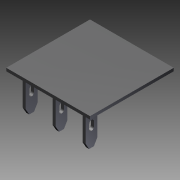
# Autodesk Inventor part: UB216KKW015C-NR
Saved by Autodesk Inventor 2015 SP1 (Build 190203100, 203)
## iProperties
Category: Electrical
Company: Autodesk Inc.
Created: 2014-12-16
Part Number: UB216KKW015C-NR
Catalog Web Link: http://www.nkkswitches.com/
Description: PC and Snap-in Mount Non-Illuminated Pushbuttons_ni_pole-Non-Illuminated Pushbuttons - Series UB2
Vendor: NKK Switches
Document SubType Name: Modeling
Designer: Autodesk Inc.
Manufacturer: NKKSWITCHES
Mass: 0.118482 g
Surface Area: 5.18676 cm^2
Volume: 0.118482 cm^3
Density: 1 g/cm^3
Material: Generic
Appearance: PSOLRGB-191-191-191
Title: UB21W01-5Cni_pole
Author: Autodesk Inc.
Comments: Non-Illuminated Pushbuttons - Series UB2
Autodesk Inventor part; units mm, degrees
sketch "Sketch_1" plane through (0, 0, 0) normal (0, 1, 0) x (-1, 0, 0)
  line L0 (7.112, -7.112) -> (7.112, 7.112)
  line L1 (7.112, 7.112) -> (-7.112, 7.112)
  line L2 (-7.112, 7.112) -> (-7.112, -7.112)
  line L3 (-7.112, -7.112) -> (7.112, -7.112)
  constraints: 8 end point
extrude "Extrusion1" add sketch "Sketch_1" along normal blind 0.508
sketch "Sketch_2" plane through (-5.08, 0, 0) normal (1, 0, 0) x (0, 0, -1)
  line L0 (-6.0833, -4.9859) -> (-5.4864, -6.0198)
  line L1 (-5.4864, -6.0198) -> (-4.6736, -6.0198)
  line L2 (-4.6736, -6.0198) -> (-4.0767, -4.9859)
  line L3 (-4.0767, -4.9859) -> (-4.0767, 0.508)
  line L4 (-4.0767, 0.508) -> (-6.0833, 0.508)
  line L5 (-6.0833, 0.508) -> (-6.0833, -4.9859)
  line L6 (-5.4864, -2.3622) -> (-5.4864, -3.1496)
  arc A0 (-5.4864, -3.1496) -> (-5.08, -3.556) centre (-5.08, -3.1496) ccw
  arc A1 (-5.08, -3.556) -> (-4.6736, -3.1496) centre (-5.08, -3.1496) ccw
  line L7 (-4.6736, -3.1496) -> (-4.6736, -2.3622)
  arc A2 (-4.6736, -2.3622) -> (-5.08, -1.9558) centre (-5.08, -2.3622) ccw
  arc A3 (-5.08, -1.9558) -> (-5.4864, -2.3622) centre (-5.08, -2.3622) ccw
  constraints: 16 end point, 8 point on circle, 4 centre point
extrude "Extrusion2" add sketch "Sketch_2" along normal mid plane 0.508
sketch "Sketch_4" plane through (0, 0, 0) normal (1, 0, 0) x (0, 1, 0)
  line L0 (-4.9859, 6.0833) -> (-6.0198, 5.4864)
  line L1 (-6.0198, 5.4864) -> (-6.0198, 4.6736)
  line L2 (-6.0198, 4.6736) -> (-4.9859, 4.0767)
  line L3 (-4.9859, 4.0767) -> (0.508, 4.0767)
  line L4 (0.508, 4.0767) -> (0.508, 6.0833)
  line L5 (0.508, 6.0833) -> (-4.9859, 6.0833)
  line L6 (-2.3622, 5.4864) -> (-3.1496, 5.4864)
  arc A0 (-3.1496, 5.4864) -> (-3.556, 5.08) centre (-3.1496, 5.08) ccw
  arc A1 (-3.556, 5.08) -> (-3.1496, 4.6736) centre (-3.1496, 5.08) ccw
  line L7 (-3.1496, 4.6736) -> (-2.3622, 4.6736)
  arc A2 (-2.3622, 4.6736) -> (-1.9558, 5.08) centre (-2.3622, 5.08) ccw
  arc A3 (-1.9558, 5.08) -> (-2.3622, 5.4864) centre (-2.3622, 5.08) ccw
  constraints: 16 end point, 8 point on circle, 4 centre point
extrude "Extrusion3" add sketch "Sketch_4" along normal mid plane 0.508
sketch "Sketch_6" plane through (5.08, 0, 0) normal (1, 0, 0) x (0, 0, -1)
  line L0 (-6.0833, -4.9859) -> (-5.4864, -6.0198)
  line L1 (-5.4864, -6.0198) -> (-4.6736, -6.0198)
  line L2 (-4.6736, -6.0198) -> (-4.0767, -4.9859)
  line L3 (-4.0767, -4.9859) -> (-4.0767, 0.508)
  line L4 (-4.0767, 0.508) -> (-6.0833, 0.508)
  line L5 (-6.0833, 0.508) -> (-6.0833, -4.9859)
  line L6 (-5.4864, -2.3622) -> (-5.4864, -3.1496)
  arc A0 (-5.4864, -3.1496) -> (-5.08, -3.556) centre (-5.08, -3.1496) ccw
  arc A1 (-5.08, -3.556) -> (-4.6736, -3.1496) centre (-5.08, -3.1496) ccw
  line L7 (-4.6736, -3.1496) -> (-4.6736, -2.3622)
  arc A2 (-4.6736, -2.3622) -> (-5.08, -1.9558) centre (-5.08, -2.3622) ccw
  arc A3 (-5.08, -1.9558) -> (-5.4864, -2.3622) centre (-5.08, -2.3622) ccw
  constraints: 16 end point, 8 point on circle, 4 centre point
extrude "Extrusion4" add sketch "Sketch_6" along normal mid plane 0.508
ref_plane "pole_to_body_XY" through (0, 0.508, 0) normal (0, 1, 0) x (1, 0, 0)
ref_plane "pole_to_body_YZ" through (0, 0.508, 0) normal (1, 0, 0) x (0, 0, -1)
ref_plane "pole_to_body_ZX" through (0, 0.508, 0) normal (0, 0, -1) x (0, 1, 0)
body "Solid1"
